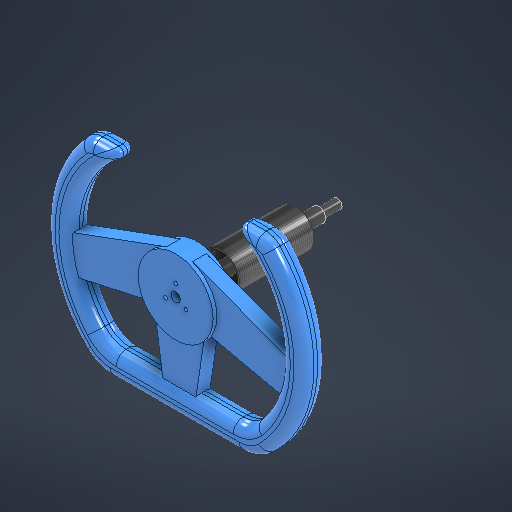
# Autodesk Inventor part: steeringwheel
Saved by Autodesk Inventor 2026.2 (Build 302298010, 298A)
## iProperties
Created: 2026-07-06
Part Number: steeringwheel
Material: Generic
Document SubType Name: Modeling
Designer: tasle
Density: 1 g/cm^3
Appearance: Default
Author: tasle
Autodesk Inventor part; units mm, degrees
ref_plane "YZ Plane" through (0, 0, 0) normal (1, 0, 0) x (0, 1, 0)
ref_plane "XZ Plane" through (0, 0, 0) normal (0, 1, 0) x (-1, 0, 0)
ref_plane "XY Plane" through (0, 0, 0) normal (0, 0, 1) x (1, 0, 0)
sketch "Sketch1" plane through (0, 0, 0) normal (0, 0, 1) x (1, 0, 0)
  circle A0 centre (0, 0) radius 138.43
  circle A1 centre (0, 0) radius 40
  line L0 (0, 0) -> (-138.43, 0)
  line L1 (0, 0) -> (-134.318, -33.4892)
  line L2 (-13.8248, 37.535) -> (-138.1829, -8.2683)
  line L3 (0, 0) -> (0, 138.43)
  line L4 (0, 0) -> (134.318, -33.4892)
  line L5 (13.8248, 37.535) -> (138.1829, -8.2683)
  line L6 (-26, -30.3974) -> (-10, -138.0683)
  line L7 (0, 0) -> (0, -138.43)
  line L8 (26, -30.3974) -> (10, -138.0683)
  line L9 (-33.6172, -21.6769) -> (-131.4213, -43.4892)
  line L10 (33.6172, -21.6769) -> (131.4213, -43.4892)
  line L11 (-84.0409, -110) -> (84.0409, -110)
  line L12 (-95.7229, 100) -> (95.7229, 100)
  circle A2 centre (0, 0) radius 113.03
  line L13 (-109.5705, -84.6) -> (109.5705, -84.6)
  circle A3 centre (0, 0) radius 5
  point P0 (0, -40)
  point P1 (-38.8118, -9.6769)
  point P2 (-52.6857, 100)
  point P3 (52.6857, 100)
  point P4 (74.9575, -84.6)
  point P5 (-74.9575, -84.6)
  point P6 (17.9454, -84.6)
  point P7 (-17.9454, -84.6)
  point P8 (113.0256, 0.9976)
  point P9 (106.4772, -37.9262)
  point P10 (-106.4772, -37.9262)
  point P11 (-113.0256, 0.9976)
  dimension "d0" = 276.86
  dimension "d1" = 80
  dimension "d2" = 14
  dimension "d3" = 26
  dimension "d4" = 10
  dimension "d5" = 10
  dimension "d6" = 12
  dimension "d7" = 100
  dimension "d8" = 110
  dimension "d9" = 226.06
  dimension "d10" = 25.4
  dimension "d11" = 10
  constraints: 28 end point, 7 symmetric about line, 5 point on circle, 4 coincident, 3 centre point, 3 horizontal, 2 point on line, 2 vertical, 1 parallel, 1 tangent, 15 other
  measures "d1" diameter of A1
  measures "d2" angle of L1 L0
  measures "d3" horizontal distance of L6.start point (0, -40)
  measures "d4" horizontal distance of L6.end L7.end
  measures "d5" vertical distance of L9.end L1.end
  measures "d6" vertical distance of point (-38.812, -9.677) L9.start
  measures "d7" distance from line of point (0, 0) L12
  measures "d8" distance from line of L11 point (0, 0)
  measures "d9" diameter of A2
  measures "d10" distance between parallel lines of L11 L13
  measures "d11" diameter of A3
extrude "Extrusion1" add sketch "Sketch1" along normal mid plane 25.4 contours A0 L5 A2 L12 | A0 L4 A2 L5 | A0 L10 A2 L4 | L12 A2 L2 L0 A0 | A0 L13 A2 L10 | L0 L2 A0 | A0 L11 A2 L13 | L2 L0 A2 L1 A0 | L2 A2 L0 | A2 L11 L8 L13 | L1 A2 L9 A0 | L8 L11 L7 L13 | L9 A2 L13 A0 | L7 L11 L6 L13 | L13 A2 L11 A0 | L6 L11 A2 L13
extrude "Extrusion2" add sketch "Sketch1" along normal mid plane 15 contours A2 L4 A1 L5 | A2 L10 A1 L4 | L2 A1 L0 A2 | L0 A1 L1 A2 | L13 L7 A1 L8 | L1 A1 L9 A2 | L13 L6 A1 L7
extrude "Extrusion3" add sketch "Sketch1" along normal mid plane 23 contours A1 L4 A3 L3 | L3 A3 L0 A1 | A1 L7 A3 L4 | L0 A3 L1 A1 | L7 A1 L1 A3
fillet "Fillet1" radius 30 2 edges at (-74.9575, -84.6, 0) (74.9575, -84.6, 0)
fillet "Fillet2" radius 40 2 edges at (-84.0409, -110, 0) (84.0409, -110, 0)
fillet "Fillet3" radius 5 2 edges at (-52.6857, 100, 0) (52.6857, 100, 0)
fillet "Fillet4" radius 20 2 edges at (-95.7229, 100, 0) (95.7229, 100, 0)
fillet "Fillet5" radius 10.7 32 edges at (-84.3996, -106.9991, 12.7) (0, -110, 12.7) (84.3996, -106.9991, 12.7) (138.3876, -3.4262, 12.7) (95.3811, 98.3058, 12.7) (78.6842, 100, 12.7) (65.2936, 96.5617, 12.7) (112.3601, 12.2876, 12.7) (74.9656, -81.9115, 12.7) (0, -84.6, 12.7) (-74.9656, -81.9115, 12.7) (-112.3601, 12.2876, 12.7) (-65.2936, 96.5617, 12.7) (-78.6842, 100, 12.7) (-95.3811, 98.3058, 12.7) (-138.3876, -3.4262, 12.7) (-95.3811, 98.3058, -12.7) (-78.6842, 100, -12.7) (-65.2936, 96.5617, -12.7) (-112.3601, 12.2876, -12.7) (-74.9656, -81.9115, -12.7) (0, -84.6, -12.7) (74.9656, -81.9115, -12.7) (112.3601, 12.2876, -12.7) (65.2936, 96.5617, -12.7) (78.6842, 100, -12.7) (95.3811, 98.3058, -12.7) (138.3876, -3.4262, -12.7) (84.3996, -106.9991, -12.7) (0, -110, -12.7) (-84.3996, -106.9991, -12.7) (-138.3876, -3.4262, -12.7)
sketch "Sketch2" plane through (0, 0, 11.5) normal (0, 0, 1) x (1, 0, 0)
  circle A0 centre (0, 0) radius 12.5
  circle A1 centre (0, 12.5) radius 2
  dimension "d25" = 25
  dimension "d26" = 4
  constraints: 1 centre point, 1 coincident, 1 vertical alignment, 2 other
  measures "d26" diameter of A1
extrude "Extrusion4" cut sketch "Sketch2" against normal blind 23 contours A1 A0 | A0 A1 picked at (0, 11.8215) picked at (0.0558, 13.1524)
pattern_circular "Circular Pattern1" count 3 over 360 about axis through (0, 0, 0) along (0, 0, 1) of "Extrusion4"
sketch "Sketch3" plane through (0, 0, -11.5) normal (0, 0, -1) x (-1, 0, 0)
  circle A0 centre (0, 0) radius 17.5
  circle A1 centre (0, 0) radius 7.5
  circle A2 centre (0, 12.5) radius 2 projected
  circle A3 centre (10.8253, -6.25) radius 2 projected
  circle A4 centre (-10.8253, -6.25) radius 2 projected
  dimension "d32" = 35
  dimension "d33" = 15
  constraints: 2 centre point, 2 coincident
  measures "d32" diameter of A0
  measures "d33" diameter of A1
extrude "Extrusion5" add sketch "Sketch3" along normal blind 5 separate body
extrude "Extrusion6" add sketch "Sketch3" along normal blind 130 contours A1 bodies 2
sketch "Sketch5" plane through (0, 0, -141.5) normal (0, 0, -1) x (-1, 0, 0)
  circle A0 centre (0, 0) radius 5
  constraints: 1 centre point, 1 coincident
extrude "Extrusion7" add sketch "Sketch5" along normal blind 20 bodies 2
ref_plane "Work Plane1" through (0, 0, -76.5) normal (0, 0, -1) x (-1, 0, 0)
sketch "Sketch6" plane through (0, 0, -76.5) normal (0, 0, -1) x (-1, 0, 0)
  circle A0 centre (0, 0) radius 20
  circle A1 centre (0, 0) radius 18.5
  circle A2 centre (0, 0) radius 5 projected
  circle A3 centre (0, 0) radius 17.5
  dimension "d41" = 40
  dimension "d42" = 37
  dimension "d43" = 35
  constraints: 3 centre point, 3 coincident
  measures "d41" diameter of A0
  measures "d42" diameter of A1
  measures "d43" diameter of A3
extrude "Extrusion8" add sketch "Sketch6" along normal mid plane 80 separate body contours A0
extrude "Extrusion9" add sketch "Sketch6" along normal mid plane 66 contours A1 bodies 3
body "Solid1"
